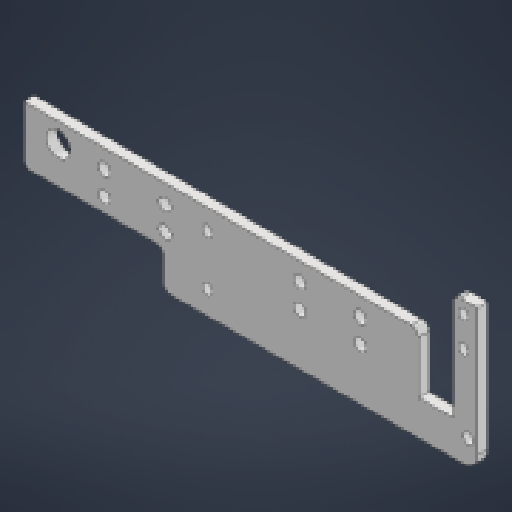
# Autodesk Inventor part: 外宽挤压
Saved by Autodesk Inventor 2025 (Build 290162000, 162)
## iProperties
Created: 2026-04-26
Part Number: 外宽挤压
Material: 常规
Document SubType Name: Modeling
Designer: XH
Density: 1 g/cm^3
Appearance: 默认
Author: XH
Autodesk Inventor part; units mm, degrees
ref_plane "YZ Plane" through (0, 0, 0) normal (1, 0, 0) x (0, 1, 0)
ref_plane "XZ Plane" through (0, 0, 0) normal (0, 1, 0) x (-1, 0, 0)
ref_plane "XY Plane" through (0, 0, 0) normal (0, 0, 1) x (1, 0, 0)
sketch "草图1" plane through (0, 0, 0) normal (0, 0, 1) x (1, 0, 0)
  line L0 (-43.79, -13.889) -> (86.21, -13.889)
  line L1 (86.21, -13.889) -> (86.21, 16.111)
  line L2 (86.21, 16.111) -> (-43.79, 16.111)
  line L3 (-43.79, 16.111) -> (-43.79, -13.889)
  dimension "d3" = 130
  dimension "d4" = 30
  constraints: 8 end point, 2 parallel, 1 horizontal, 1 perpendicular
  measures "d3" distance of L0.start L0.end
  measures "d4" distance of L0.end L1.end
extrude "拉伸1" add sketch "草图1" along normal blind 3
sketch "草图2" plane through (0, 0, 3) normal (0, 0, 1) x (1, 0, 0)
  line L0 (86.21, 16.111) -> (-43.79, 16.111) projected
  line L1 (69.2643, 16.111) -> (79.2643, 16.111)
  line L2 (79.2643, 16.111) -> (79.2643, -3.889)
  line L3 (79.2643, -3.889) -> (69.2643, -3.889)
  line L4 (69.2643, -3.889) -> (69.2643, 16.111)
  point P0 (0, 0)
  dimension "d5" = 10
  dimension "d6" = 20
  constraints: 8 end point, 2 parallel, 1 horizontal, 1 perpendicular, 1 point on line
  measures "d5" distance of L2.end L3.end
  measures "d6" distance of L1.end L2.end
extrude "拉伸2" cut sketch "草图2" against normal blind 3
fillet "圆角1" radius 2 2 edges at (69.2643, 16.111, 1.5) (79.2643, 16.111, 1.5)
sketch "草图3" plane through (0, 0, 3) normal (0, 0, 1) x (1, 0, 0)
  line L0 (-43.79, 16.111) -> (-43.79, -13.889) projected
  line L1 (-43.79, -13.889) -> (-3.79, -13.889)
  line L2 (-3.79, -13.889) -> (-3.79, 4.111)
  line L3 (-3.79, 4.111) -> (-43.79, 4.111)
  line L4 (-43.79, 4.111) -> (-43.79, -13.889)
  point P0 (0, 0)
  dimension "d10" = 40
  dimension "d11" = 18
  constraints: 8 end point, 2 parallel, 1 horizontal, 1 perpendicular
  measures "d10" distance between parallel lines of L2 L0
  measures "d11" distance between parallel lines of L1 L3
extrude "拉伸3" cut sketch "草图3" against normal blind 3
fillet "圆角2" radius 2 2 edges at (-3.79, 4.111, 1.5) (-3.79, -13.889, 1.5)
fillet "圆角3" radius 2 1 edges at (-43.79, 4.111, 1.5)
move faces "移动1" translate (0, 10.75, 0) faces at (84.5614, 16.111, 1)
fillet "圆角4" radius 4.25 1 edges at (86.21, -13.889, 1.5)
move faces "移动2" translate (0, -7.25, 0) faces at (-17.79, 4.111, 1)
sketch "草图4" plane through (0, 0, 0) normal (0, 0, -1) x (-1, 0, 0)
  line L0 (-0.892, -15.4705) -> (-0.8856, 17.0295) projected
  line L1 (-16.692, -15.4674) -> (-16.6856, 17.0326) projected
  line L2 (-0.889, 0) -> (-16.689, 0.0031)
  line L3 (-8.789, -13.6529) -> (-8.789, 16.111)
  line L4 (-67.2643, 16.111) -> (43.79, 16.111) projected
  circle A0 centre (-8.789, -7.1669) radius 1.55
  circle A1 centre (-8.7862, 7.17) radius 1.55
  point P0 (0, 0)
  point P1 (-8.789, 0.0016)
  dimension "d23" = 3.1
  constraints: 5 point on line, 4 end point, 2 centre point, 1 midpoint, 1 perpendicular, 1 symmetric about line, 1 vertical, 1 other
  measures "d23" diameter of A0
extrude "拉伸4" cut sketch "草图4" against normal blind 10 contours A1 L3 | L3 A1 | A0 L3 | L3 A0
sketch "草图5" plane through (0, 0, 0) normal (0, 0, -1) x (-1, 0, 0)
  circle A0 centre (-83.46, -6.8603) radius 1.5 projected
  circle A1 centre (-82.1717, 14.6045) radius 1.5 projected
  circle A2 centre (-82.1717, 23.2524) radius 1.5 projected
  line L0 (-67.41, 27.075) -> (-67.41, 17.075) projected
  line L1 (-86.21, 27.075) -> (-67.41, 27.075) projected
  line L2 (-86.21, -11.1435) -> (-86.21, 27.075) projected
  line L3 (-80.71, -11.1435) -> (-86.21, -11.1435) projected
  line L4 (-80.71, 10.8565) -> (-80.71, -11.1435) projected
  line L5 (-77.71, 10.8565) -> (-80.71, 10.8565) projected
  line L6 (-77.71, 25.075) -> (-77.71, 10.8565) projected
  line L7 (-72.41, 25.075) -> (-77.71, 25.075) projected
  line L8 (-72.41, 17.075) -> (-72.41, 25.075) projected
  line L9 (-67.41, 17.075) -> (-72.41, 17.075) projected
  point P0 (0, 0)
extrude "拉伸5" cut sketch "草图5" against normal blind 10 contours A0 | A1 | A2
sketch "草图6" plane through (0, 0, 3) normal (0, 0, 1) x (1, 0, 0)
  line L0 (-43.79, 16.111) -> (-43.79, -1.139) projected
  line L1 (-43.79, 7.486) -> (-28.8544, 7.486)
  circle A0 centre (-33.8796, 7.486) radius 3.5
  point P0 (0, 0)
  dimension "d28" = 7
  constraints: 2 end point, 1 centre point, 1 horizontal, 1 midpoint, 1 point on line
  measures "d28" diameter of A0
extrude "拉伸6" cut sketch "草图6" against normal blind 10
move faces "移动3" translate (0, -3, 0) faces at (30.2462, 16.111, 1)
sketch "草图7" plane through (0, 0, 3) normal (0, 0, 1) x (1, 0, 0)
  line L0 (-24.0337, 11.8662) -> (-17.4166, 11.868) projected
  line L1 (-24.0308, -3.1293) -> (-24.0337, 11.8662) projected
  line L2 (-17.4137, -3.1275) -> (-24.0308, -3.1293) projected
  line L3 (-17.4166, 11.868) -> (-17.4137, -3.1275) projected
  line L4 (-0.0338, 11.8727) -> (-6.6509, 11.8709) projected
  line L5 (-6.648, -3.1245) -> (-6.6509, 11.8709) projected
  line L6 (-6.648, -3.1245) -> (-0.0309, -3.1227) projected
  line L7 (-0.0309, -3.1227) -> (-0.0338, 11.8727) projected
  line L8 (31.8924, 11.8777) -> (38.5095, 11.8792) projected
  line L9 (31.8954, -3.1177) -> (31.8924, 11.8777) projected
  line L10 (38.5125, -3.1162) -> (31.8954, -3.1177) projected
  line L11 (38.5095, 11.8792) -> (38.5125, -3.1162) projected
  line L12 (55.8954, -3.1123) -> (55.8924, 11.8832) projected
  line L13 (55.8924, 11.8832) -> (49.2753, 11.8817) projected
  line L14 (49.2783, -3.1138) -> (49.2753, 11.8817) projected
  line L15 (49.2783, -3.1138) -> (55.8954, -3.1123) projected
  line L16 (55.8954, -3.1123) -> (55.8924, 11.8832) projected
  line L17 (-20.7252, 11.8671) -> (-20.7222, -3.1284)
  line L18 (-3.3424, 11.8718) -> (-3.3394, -3.1236)
  line L19 (35.201, 11.8785) -> (35.2039, -3.117)
  line L20 (52.5838, 11.8824) -> (52.5868, -3.113)
  circle A0 centre (-20.7244, 7.7585) radius 1.75
  line L21 (-24.0323, 4.3685) -> (-17.4152, 4.3703)
  circle A1 centre (-20.7225, 0.9802) radius 1.75
  circle A2 centre (-3.3416, 7.7585) radius 1.75
  circle A3 centre (-3.3402, 0.9802) radius 1.75
  circle A4 centre (52.586, 0.9802) radius 1.75
  circle A5 centre (52.5847, 7.7585) radius 1.75
  circle A6 centre (35.2031, 0.9802) radius 1.75
  circle A7 centre (35.2018, 7.7585) radius 1.75
  ellipse E0 centre (-20.7337, 7.8342) end of major axis (-18.9969, 8.0485) minor radius 1.7489 projected
  ellipse E1 centre (-20.7324, 1.06) end of major axis (-18.9956, 1.2743) minor radius 1.7489 projected
  ellipse E2 centre (-3.3511, 7.8355) end of major axis (-1.6143, 8.0498) minor radius 1.7489 projected
  ellipse E3 centre (-3.3502, 1.0613) end of major axis (-1.6134, 1.2756) minor radius 1.7489 projected
  ellipse E4 centre (52.5752, 7.8461) end of major axis (54.3187, 7.9959) minor radius 1.7489 projected
  ellipse E5 centre (52.576, 1.0719) end of major axis (54.3196, 1.2217) minor radius 1.7489 projected
  ellipse E6 centre (35.1924, 7.8455) end of major axis (36.936, 7.9954) minor radius 1.7489 projected
  ellipse E7 centre (35.1938, 1.0714) end of major axis (36.9374, 1.2212) minor radius 1.7489 projected
  point P0 (0, 0)
  dimension "d34" = 3.5
  dimension "d35" = 3.5
  dimension "d37" = 3.5
  dimension "d38" = 3.5
  constraints: 10 end point, 10 midpoint, 8 centre point, 7 point on line, 6 horizontal alignment, 1 symmetric about line, 1 other
  measures "d34" diameter of A0
  measures "d35" diameter of A2
  measures "d37" diameter of A5
  measures "d38" diameter of A7
extrude "拉伸7" cut sketch "草图7" against normal blind 10 contours A0 E0 L17 | L17 E0 A0 | A0 L17 E0 | E0 L17 A0 | A1 E1 L17 | L17 E1 A1 | A1 E1 L17 | L17 E1 A1 | A2 E2 L18 | L18 E2 A2 | A2 L18 E2 | E2 L18 A2 | A3 E3 L18 | L18 E3 A3 | E3 A3 L18 | L18 A3 E3 | A7 E6 L19 | L19 E6 A7 | A7 L19 E6 | E6 L19 A7 | A6 E7 L19 | L19 E7 A6 | E7 A6 L19 | L19 A6 E7 | A4 E5 L20 | L20 E5 A4 | E5 A4 L20 | L20 A4 E5 | A5 E4 L20 | L20 E4 A5 | A5 L20 E4 | E4 L20 A5 picked at (-20.5926, 7.2422) picked at (-20.8624, 8.3509) picked at (-20.4626, 6.0902) picked at (-20.8656, 6.0515) picked at (-20.8642, -0.7254) picked at (-20.4612, -0.6854) picked at (-20.5912, 0.4666) picked at (-20.861, 1.5739) picked at (-3.2098, 7.2431) picked at (-3.4796, 8.3513) picked at (-3.0798, 6.0911) picked at (-3.4828, 6.0519) picked at (-3.4816, -0.725) picked at (-3.0784, -0.6845) picked at (-3.4782, 1.5744) picked at (-3.2085, 0.4675) picked at (35.3448, 7.2525) picked at (35.0652, 8.355) picked at (35.8749, 6.2153) picked at (35.0589, 6.0557) picked at (35.0596, -0.721) picked at (35.4761, -0.675) picked at (35.0671, 1.5782) picked at (35.3461, 0.477) picked at (52.4431, -0.721) picked at (52.859, -0.6746) picked at (52.4494, 1.5783) picked at (52.7289, 0.4774) picked at (52.7276, 7.2529) picked at (52.4481, 8.3552) picked at (53.2577, 6.2157) picked at (52.4417, 6.0559)
